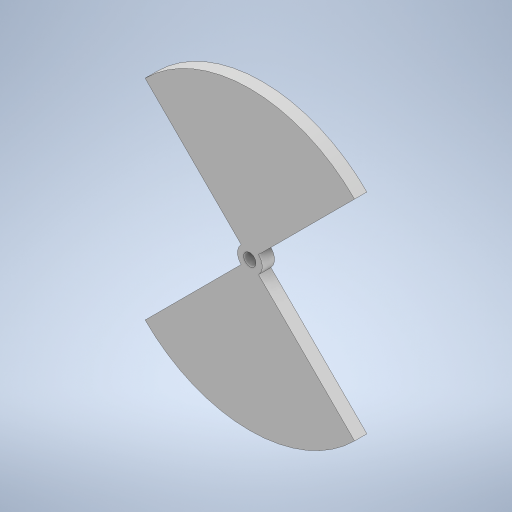
# Autodesk Inventor part: Release2
Saved by Autodesk Inventor 2024 (Build 280153000, 153)
## iProperties
Created: 2023-11-02
Part Number: Release2
Material: Generic
Document SubType Name: Modeling
Designer: flynf
Density: 1 g/cm^3
Appearance: Default
Author: flynf
Autodesk Inventor part; units mm, degrees
ref_plane "YZ Plane" through (0, 0, 0) normal (1, 0, 0) x (0, 1, 0)
ref_plane "XZ Plane" through (0, 0, 0) normal (0, 1, 0) x (-1, 0, 0)
ref_plane "XY Plane" through (0, 0, 0) normal (0, 0, 1) x (1, 0, 0)
sketch "Sketch1" plane through (0, 0, 0) normal (0, 0, 1) x (1, 0, 0)
  line L0 (-2.2451, -2.2451) -> (-26.9408, -26.9408)
  line L1 (2.2451, -2.2451) -> (26.9408, -26.9408)
  line L2 (2.2451, 2.2451) -> (26.9408, 26.9408)
  line L3 (-2.2451, 2.2451) -> (-26.9408, 26.9408)
  circle A0 centre (0, 0) radius 1.5875
  arc A1 (2.2451, -2.2451) -> (2.2451, 2.2451) centre (0, 0) ccw
  arc A2 (-2.2451, 2.2451) -> (-2.2451, -2.2451) centre (0, 0) ccw
  line L4 (0, 0) -> (-1.5875, 0)
  arc A3 (26.9408, 26.9408) -> (-26.9408, 26.9408) centre (0, 0) ccw
  arc A4 (-26.9408, -26.9408) -> (26.9408, -26.9408) centre (0, 0) ccw
  dimension "d5" = 3.175
  dimension "d1" = 90
  dimension "d2" = 90
  dimension "d3" = 90
  constraints: 10 end point, 8 point on circle, 4 centre point, 3 coincident, 1 horizontal, 1 horizontal alignment, 2 other
  measures "d1" angle of L3 L2
  measures "d2" angle of L0 L1
  measures "d3" angle of L2 L1
extrude "Extrusion1" add sketch "Sketch1" along normal blind 3.175
body "Solid1"
